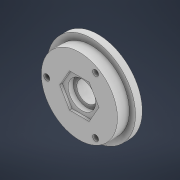
# Autodesk Inventor part: Planet_Carrier_Mid
Saved by Autodesk Inventor 2021 (Build 250183000, 183)
## iProperties
Created: 2025-03-15
Part Number: Planet_Carrier_Mid
Material: Generic
Document SubType Name: Modeling
Designer: rocke
Density: 0.450533 g/cm^3
Appearance: Default
Mass: 8.63 g
Surface Area: 64.1791 cm^2
Volume: 19.1551 cm^3
3D_PRINTED: True
Author: rocke
Autodesk Inventor part; units mm, degrees
ref_plane "YZ Plane" through (0, 0, 0) normal (1, 0, 0) x (0, 1, 0)
ref_plane "XZ Plane" through (0, 0, 0) normal (0, 1, 0) x (-1, 0, 0)
sketch "Sketch1" plane through (0, 0, 0) normal (0, 0, 1) x (1, 0, 0)
  circle A0 centre (0, 0) radius 22.4
  dimension "d0" = 44.8
  constraints: 1 centre point, 1 coincident
  measures "d0" diameter of A0
extrude "Extrusion1" add sketch "Sketch1" along normal blind 11
sketch "Sketch8" plane through (0, 0, 0) normal (0, 0, -1) x (-1, 0, 0)
  circle A0 centre (0, 0) radius 26
  dimension "d23" = 52
  constraints: 1 centre point, 1 coincident
  measures "d23" diameter of A0
extrude "Extrusion7" add sketch "Sketch8" against normal blind 4
sketch "Sketch2" plane through (0, 0, 0) normal (0, 0, -1) x (-1, 0, 0)
  circle A0 centre (19.155, 0) radius 1.75
  circle A1 centre (-9.5775, 16.5887) radius 1.75
  circle A2 centre (-9.5775, -16.5887) radius 1.75
  point P0 (0, 0)
  dimension "d3" = 3.5
  dimension "d4" = 19.155
  dimension "d7" = 360
  constraints: 3 centre point, 7 other
  measures "d3" diameter of A0
  measures "d4" distance of A0.centre point (0, 0)
extrude "Extrusion2" cut sketch "Sketch2" against normal through all
sketch "Sketch3" plane through (0, 0, 11) normal (0, 0, 1) x (1, 0, 0)
  circle A0 centre (0, 0) radius 6
  dimension "d11" = 12
  constraints: 1 centre point, 1 coincident
  measures "d11" diameter of A0
extrude "Extrusion3" cut sketch "Sketch3" against normal blind 2
sketch "Sketch4" plane through (0, 0, 11) normal (0, 0, 1) x (1, 0, 0)
  circle A0 centre (0, 0) radius 6 projected
  line L0 (11.547, 0) -> (5.7735, -10)
  line L1 (5.7735, -10) -> (-5.7735, -10)
  line L2 (-5.7735, -10) -> (-11.547, 0)
  line L3 (-11.547, 0) -> (-5.7735, 10)
  line L4 (-5.7735, 10) -> (5.7735, 10)
  line L5 (5.7735, 10) -> (11.547, 0)
  circle A1 centre (0, 0) radius 6
  dimension "d14" = 10
  constraints: 12 end point, 2 coincident, 1 centre point, 1 concentric, 1 horizontal, 13 other
  measures "d14" distance from line of L4 point (0, 0)
extrude "Extrusion4" cut sketch "Sketch4" against normal blind 1.5
sketch "Sketch5" plane through (0, 0, 0) normal (0, 0, -1) x (-1, 0, 0)
  line L0 (5.7735, 10) -> (-5.7735, 10) projected
  line L1 (-5.7735, 10) -> (5.7735, 10)
  line L2 (5.7735, 10) -> (11.547, 0)
  line L3 (11.547, 0) -> (5.7735, -10)
  line L4 (5.7735, -10) -> (-5.7735, -10)
  line L5 (-5.7735, -10) -> (-11.547, 0)
  line L6 (-11.547, 0) -> (-5.7735, 10)
  point P0 (0, 0)
  point P1 (0, 0)
  constraints: 12 end point, 1 coincident, 13 other
extrude "Extrusion5" add sketch "Sketch5" along normal blind 1.5
ref_plane "Work Plane1" through (0, 0, 4.5) normal (0, 0, 1) x (1, 0, 0)
sketch "Sketch6" plane through (0, 0, 4.5) normal (0, 0, 1) x (1, 0, 0)
  circle A0 centre (0, 0) radius 22.6071
  circle A1 centre (0, 0) radius 21.1
  dimension "d20" = 42.2
  constraints: 2 centre point, 2 coincident
  measures "d20" diameter of A1
extrude "Extrusion6" [suppressed]
sketch "Sketch7" plane through (0, 0, 0) normal (0, 0, -1) x (-1, 0, 0)
  point P0 (0, 0)
sketch "Sketch9" plane through (0, 0, 9.5) normal (0, 0, 1) x (1, 0, 0)
  circle A0 centre (0, 0) radius 6 projected
  circle A1 centre (0, 0) radius 8.1
  dimension "d26" = 16.2
  constraints: 1 centre point, 1 coincident
  measures "d26" diameter of A1
extrude "Extrusion8" cut sketch "Sketch9" against normal blind 3 contours A0 | A1
sketch "Sketch10" plane through (0, 0, 6.5) normal (0, 0, 1) x (1, 0, 0)
  circle A0 centre (0, 0) radius 6
  dimension "d29" = 12
  constraints: 1 centre point, 1 coincident
  measures "d29" diameter of A0
extrude "Extrusion9" cut sketch "Sketch10" against normal through all
body "Solid1"
